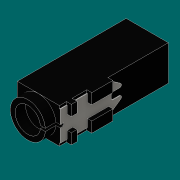
# Autodesk Inventor part: SJ-4351X-SMT
Saved by Autodesk Inventor 2016 (Build 200138000, 138)
## iProperties
Created: 2015-08-17
Part Number: SJ-4351X-SMT
Material: ABS Plastic
Document SubType Name: Modeling
Designer: Cosmic
Density: 1.06 g/cm^3
Appearance: Smooth - Black
Author: Cosmic
Autodesk Inventor part; units mm, degrees
ref_plane "YZ Plane" through (0, 0, 0) normal (1, 0, 0) x (0, 1, 0)
ref_plane "XZ Plane" through (0, 0, 0) normal (0, 1, 0) x (-1, 0, 0)
ref_plane "XY Plane" through (0, 0, 0) normal (0, 0, 1) x (1, 0, 0)
sketch "Sketch1" plane through (0, 0, 0) normal (0, 0, 1) x (1, 0, 0)
  line L0 (3, -7.75) -> (-3, -7.75)
  line L1 (-3, -7.75) -> (-3, 7.75)
  line L2 (-3, 7.75) -> (3, 7.75)
  line L3 (3, 7.75) -> (3, -7.75)
  line L4 (3, -7.75) -> (-3, 7.75) construction
  line L5 (-3, -7.75) -> (3, 7.75) construction
  point P0 (0, 0)
  dimension "d0" = 6
  dimension "d1" = 15.5
  constraints: 12 end point, 2 midpoint, 2 parallel, 1 horizontal, 1 perpendicular
  measures "d0" distance of L1.end L2.end
  measures "d1" distance of L0.end L1.end
extrude "Extrusion1" add sketch "Sketch1" along normal blind 5
sketch "Sketch2" plane through (-3, -7.75, 0) normal (0, -1, 0) x (1, 0, 0)
  line L0 (6, 0) -> (0, 0) projected
  line L1 (6, 0) -> (6, 5) projected
  line L2 (0, 5) -> (6, 5) projected
  line L3 (0, 0) -> (0, 5) projected
  line L4 (6, 0) -> (0, 0) projected
  line L5 (0, 0) -> (6, 5)
  circle A0 centre (3, 2.5) radius 2.5
  circle A1 centre (3, 2.5) radius 1.8
  point P0 (3, 0)
  dimension "d4" = 5
  dimension "d5" = 3.6
  constraints: 2 centre point, 2 end point, 1 coincident, 1 midpoint
  measures "d4" diameter of A0
  measures "d5" diameter of A1
extrude "Extrusion2" add sketch "Sketch2" along normal blind 1.5 contours A0 L5 A1 | A0 L5 A1
sketch "Sketch3" plane through (0, 0, 0) normal (0, 0, -1) x (-1, 0, 0)
  line L0 (-3, -7.75) -> (0, -7.75) projected
  line L1 (0, -7.75) -> (3, -7.75) projected
  line L2 (3, -7.75) -> (3, 7.75) projected
  line L3 (3, 7.75) -> (-3, 7.75) projected
  line L4 (-3, 7.75) -> (-3, -7.75) projected
  circle A0 centre (0, -3.25) radius 0.75
  circle A1 centre (0, 3.75) radius 0.75
  point P0 (0, 0)
  dimension "d8" = 1.5
  dimension "d9" = 1.5
  dimension "d10" = 4.5
  dimension "d11" = 7
  constraints: 2 centre point
  measures "d8" diameter of A1
  measures "d9" diameter of A0
  measures "d10" distance from line of L0 A0.centre
  measures "d11" distance of A1.centre A0.centre
extrude "Extrusion3" add sketch "Sketch3" along normal blind 0.8 contours A0 | A1
fillet "Fillet1" radius 0.2 2 edges at (0.75, -3.25, -0.8) (0.75, 3.75, -0.8)
sketch "Sketch4" plane through (3, -7.75, 0) normal (1, 0, 0) x (0, 0, -1)
  line L0 (0, 15.5) -> (0, 0) projected
  line L1 (0, 15.5) -> (-5, 15.5) projected
  line L2 (-5, 0) -> (-5, 15.5) projected
  line L3 (0, 0) -> (-5, 0) projected
  line L4 (-5, 15.5) -> (-5, 0) projected
  line L5 (-5, 1) -> (-3.5, 1)
  line L6 (-3.5, 1) -> (-3.5, 1.8)
  line L7 (-3.5, 1.8) -> (-5, 1.8)
  line L8 (-5, 1.8) -> (-5, 1)
  line L9 (0, 1) -> (-1.5, 1)
  line L10 (-1.5, 1) -> (-1.5, 1.8)
  line L11 (-1.5, 1.8) -> (0, 1.8)
  line L12 (0, 1.8) -> (0, 1)
  line L13 (-5, 3.9) -> (-3.5, 3.9)
  line L14 (-3.5, 3.9) -> (-3.5, 6.9)
  line L15 (-3.5, 6.9) -> (-5, 6.9)
  line L16 (-5, 6.9) -> (-5, 3.9)
  line L17 (0, 3.9) -> (-1.5, 3.9)
  line L18 (-1.5, 3.9) -> (-1.5, 6.9)
  line L19 (-1.5, 6.9) -> (0, 6.9)
  line L20 (0, 6.9) -> (0, 3.9)
  point P0 (0, 7.75)
  dimension "d15" = 1
  dimension "d16" = 0.8
  dimension "d17" = 1.5
  dimension "d18" = 1.5
  dimension "d19" = 1.5
  dimension "d20" = 1.5
  dimension "d21" = 3.9
  dimension "d22" = 3
  constraints: 32 end point, 8 parallel, 5 point on line, 4 horizontal, 4 perpendicular, 3 collinear
  measures "d15" distance between parallel lines of L3 L5
  measures "d16" distance of L5.end L6.end
  measures "d17" distance between parallel lines of L4 L6
  measures "d18" distance between parallel lines of L12 L10
  measures "d19" distance between parallel lines of L2 L14
  measures "d20" distance between parallel lines of L20 L18
  measures "d21" distance between parallel lines of L3 L17
  measures "d22" distance between parallel lines of L17 L19
extrude "Extrusion4" add sketch "Sketch4" along normal blind 0.7 contours L0 L17 L18 L19 | L15 L14 L13 L2 | L0 L9 L10 L11 | L7 L6 L5 L2
sketch "Sketch5" plane through (3, 7.75, 5) normal (1, 0, 0) x (0, 0, -1)
  line L0 (3.5, -8.6) -> (5, -8.6) projected
  line L1 (5, 0) -> (5, -8.6) projected
  line L2 (5, 0) -> (0, 0) projected
  line L3 (0, -8.6) -> (0, 0) projected
  line L4 (0, -8.6) -> (1.5, -8.6) projected
  line L5 (1.5, -8.6) -> (1.5, -11.6) projected
  line L6 (1.5, -11.6) -> (0, -11.6) projected
  line L7 (0, -13.7) -> (0, -11.6) projected
  line L8 (0, -13.7) -> (1.5, -13.7) projected
  line L9 (1.5, -13.7) -> (1.5, -14.5) projected
  line L10 (1.5, -14.5) -> (0, -14.5) projected
  line L11 (0, -15.5) -> (0, -14.5) projected
  line L12 (5, -15.5) -> (0, -15.5) projected
  line L13 (5, -14.5) -> (5, -15.5) projected
  line L14 (5, -14.5) -> (3.5, -14.5) projected
  line L15 (3.5, -14.5) -> (3.5, -13.7) projected
  line L16 (3.5, -13.7) -> (5, -13.7) projected
  line L17 (5, -11.6) -> (5, -13.7) projected
  line L18 (5, -11.6) -> (3.5, -11.6) projected
  line L19 (3.5, -11.6) -> (3.5, -8.6) projected
  line L20 (0.4, -15.5) -> (0.4, -8.5)
  line L21 (0, -8.6) -> (1.5, -8.6) projected
  line L22 (0.4, -8.5) -> (1.5452, -6.8645)
  line L23 (2, -7.0079) -> (2, -7.965)
  line L24 (2.25, -8.215) -> (2.75, -8.215)
  line L25 (3, -7.965) -> (3, -7.0079)
  line L26 (3.4548, -6.8645) -> (4.6, -8.5)
  line L27 (4.6, -8.5) -> (4.6, -15.5)
  line L28 (5, -15.5) -> (0, -15.5) projected
  line L29 (2.5, -15.5) -> (2.5, 0)
  line L30 (5, 0) -> (0, 0) projected
  arc A0 (3.4548, -6.8645) -> (3, -7.0079) centre (3.25, -7.0079) ccw
  arc A1 (2, -7.0079) -> (1.5452, -6.8645) centre (1.75, -7.0079) ccw
  arc A2 (2, -7.965) -> (2.25, -8.215) centre (2.25, -7.965) ccw
  arc A3 (2.75, -8.215) -> (3, -7.965) centre (2.75, -7.965) ccw
  point P0 (5, -7.75)
  point P1 (2, -8.215)
  point P2 (3, -8.215)
  point P3 (3, -6.215)
  point P4 (2.5, -8.215)
  dimension "d25" = 0.4
  dimension "d26" = 0.4
  dimension "d27" = 145
  dimension "d28" = 145
  dimension "d29" = 1
  dimension "d30" = 7
  dimension "d31" = 7
  dimension "d32" = 2
  dimension "d33" = 0.25
  constraints: 16 end point, 9 point on line, 8 point on circle, 8 tangent, 4 centre point, 4 perpendicular, 3 equal radius, 3 midpoint, 1 parallel
  measures "d25" distance between parallel lines of L11 L20
  measures "d26" distance between parallel lines of L13 L27
  measures "d27" angle of L27 L26
  measures "d28" angle of L20 L22
  measures "d29" distance of point (2, -8.215) point (3, -8.215)
  measures "d30" distance of L20.start L20.end
  measures "d31" distance of L26.end L27.end
  measures "d32" distance from line of point (3, -6.215) L24
  measures "d33" radius of A0
extrude "Extrusion5" add sketch "Sketch5" along normal blind 0.1 contours L19 L18 L27 L16 L15 L14 L12 L29 L24 A3 L25 A0 L26 L0 | L0 L27 L18 L19 | L27 L14 L15 L16 | L29 L12 L20 L10 L9 L8 L6 L5 L4 L22 A1 L23 A2 L24 | L4 L5 L6 L20 | L20 L8 L9 L10
sketch "Sketch6" plane through (0, -9.25, 2.5) normal (0, -1, 0) x (1, 0, 0)
  circle A0 centre (0, 0) radius 1.8 projected
  circle A1 centre (0, 0) radius 2.5 projected
  line L0 (1.5, -0.2) -> (3.5, -0.2)
  line L1 (3.5, -0.2) -> (3.5, 0.2)
  line L2 (3.5, 0.2) -> (1.5, 0.2)
  line L3 (1.5, 0.2) -> (1.5, -0.2)
  line L4 (1.5, -0.2) -> (3.5, 0.2) construction
  line L5 (3.5, -0.2) -> (1.5, 0.2) construction
  point P0 (0, -2.5)
  point P1 (2.5, 0)
  dimension "d36" = 2
  dimension "d37" = 0.4
  constraints: 12 end point, 2 midpoint, 2 parallel, 1 horizontal, 1 horizontal alignment, 1 perpendicular, 1 other
  measures "d36" distance of L2.end L1.end
  measures "d37" distance of L1.end L0.end
extrude "Extrusion6" cut sketch "Sketch6" against normal blind 2 contours A0 L0 L3 L2 | A0 L2 A1 L0 | L2 L1 L0 A1 picked at (1.6, 0) picked at (2.0301, 0.1112)
equation "\"d18\" = d17"
equation "\"d19\" = d17"
equation "\"d20\" = d18"
equation "\"d26\" = d25"
equation "\"d31\" = d30"
body "Solid1"
